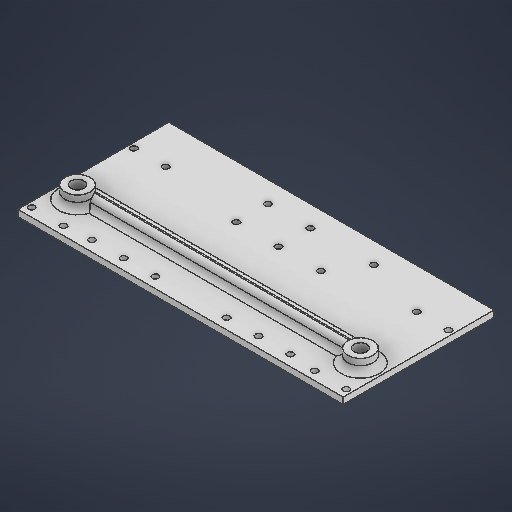
# Autodesk Inventor part: rigid_support1
Saved by Autodesk Inventor 2026.1 (Build 301233000, 233)
## iProperties
Created: 2025-10-27
Part Number: rigid_support1
Material: Generic
Document SubType Name: Modeling
Designer: emanuel
Density: 1 g/cm^3
Appearance: Default
Author: emanuel
Autodesk Inventor part; units mm, degrees
ref_plane "YZ Plane" through (0, 0, 0) normal (1, 0, 0) x (0, 1, 0)
ref_plane "XZ Plane" through (0, 0, 0) normal (0, 1, 0) x (-1, 0, 0)
ref_plane "XY Plane" through (0, 0, 0) normal (0, 0, 1) x (1, 0, 0)
sketch "Sketch1" plane through (0, 0, 0) normal (0, 1, 0) x (-1, 0, 0)
  line L0 (0, 0) -> (15, 0)
  line L1 (15, 0) -> (15, -48.3)
  line L2 (15, -48.3) -> (0, -48.3)
  line L3 (0, -48.3) -> (0, 0)
  circle A0 centre (15, 0) radius 1.5
  circle A1 centre (0, 0) radius 1.5
  circle A2 centre (15, -48.3) radius 1.5
  circle A3 centre (0, -48.3) radius 1.5
  line L4 (15, 0) -> (17.5, 0)
  line L5 (17.5, 0) -> (17.5, 4)
  line L6 (17.5, 4) -> (15, 4)
  line L7 (15, 4) -> (15, 0)
  line L8 (0, -48.3) -> (-2.5, -48.3)
  line L9 (-2.5, -48.3) -> (-2.5, -52.3)
  line L10 (-2.5, -52.3) -> (0, -52.3)
  line L11 (0, -52.3) -> (0, -48.3)
  line L12 (-2.5, -52.3) -> (17.5, -52.3)
  line L13 (17.5, -52.3) -> (17.5, 4)
  line L14 (17.5, 4) -> (-2.5, 4)
  line L15 (-2.5, 4) -> (-2.5, -52.3)
  line L16 (17.5, -26) -> (17.5, 4)
  line L17 (17.5, -44.8) -> (17.5, 4)
  line L18 (-2.5, -52.3) -> (-59.35, -52.3)
  line L19 (-2.5, -44.8) -> (-2.5, -52.3)
  line L20 (-2.5, 4) -> (-59.35, 4)
  line L21 (-59.35, 4) -> (-59.35, -52.3)
  line L22 (-59.35, -52.3) -> (-2.5, -52.3)
  line L23 (-2.5, -52.3) -> (-2.5, 4)
  line L24 (-118.7, 0) -> (-133.7, 0)
  line L25 (-133.7, 0) -> (-133.7, -48.3)
  line L26 (-133.7, -48.3) -> (-118.7, -48.3)
  line L27 (-118.7, -48.3) -> (-118.7, 0)
  circle A4 centre (-133.7, 0) radius 1.5
  circle A5 centre (-118.7, 0) radius 1.5
  circle A6 centre (-133.7, -48.3) radius 1.5
  circle A7 centre (-118.7, -48.3) radius 1.5
  line L28 (-133.7, 0) -> (-136.2, 0)
  line L29 (-136.2, 0) -> (-136.2, 4)
  line L30 (-136.2, 4) -> (-133.7, 4)
  line L31 (-133.7, 4) -> (-133.7, 0)
  line L32 (-118.7, -48.3) -> (-116.2, -48.3)
  line L33 (-116.2, -48.3) -> (-116.2, -52.3)
  line L34 (-116.2, -52.3) -> (-118.7, -52.3)
  line L35 (-118.7, -52.3) -> (-118.7, -48.3)
  line L36 (-116.2, -52.3) -> (-136.2, -52.3)
  line L37 (-136.2, -52.3) -> (-136.2, 4)
  line L38 (-136.2, 4) -> (-116.2, 4)
  line L39 (-116.2, 4) -> (-116.2, -52.3)
  line L40 (-136.2, -26) -> (-136.2, 4)
  line L41 (-136.2, -44.8) -> (-136.2, 4)
  line L42 (-116.2, -52.3) -> (-59.35, -52.3)
  line L43 (-116.2, -44.8) -> (-116.2, -52.3)
  line L44 (-116.2, 4) -> (-59.35, 4)
  line L45 (-59.35, -52.3) -> (-116.2, -52.3)
  line L46 (-116.2, -52.3) -> (-116.2, 4)
  point P0 (0, -52.3)
  point P1 (16.5, 0)
  point P2 (15, 1.5)
  dimension "d0" = 15
  dimension "d1" = 48.3
  dimension "d2" = 3
  dimension "d3" = 3
  dimension "d4" = 3
  dimension "d5" = 3
  dimension "d6" = 2.5
  dimension "d7" = 4
  dimension "d8" = 2.5
  dimension "d9" = 4
  dimension "d87" = 56.85
  constraints: 94 end point, 20 symmetric about line, 10 parallel, 8 centre point, 8 coincident, 6 horizontal, 5 perpendicular, 4 other
  measures "d0" distance of L1.end L2.end
  measures "d1" distance of L0.end L1.end
  measures "d2" diameter of A0
  measures "d3" diameter of A1
  measures "d4" diameter of A2
  measures "d5" diameter of A3
  measures "d6" distance of L6.end L5.end
  measures "d7" distance of L5.end L4.end
  measures "d8" distance of L10.end L9.end
  measures "d9" distance of L9.end L8.end
  measures "d87" distance of L9.end L18.end
extrude "Extrusion1" add sketch "Sketch1" along normal blind 3 contours A1 L3 A3 L8 L15 L14 L7 A0 L0 | L0 A0 L1 A2 L2 A3 L3 A1 | L7 L6 L5 L4 A0 | A0 L4 L13 L12 L11 A3 L2 A2 L1 | A3 L11 L10 L9 L8 | L9 L18 L21 L20 L15 | L21 L42 L33 L39 L44 | L39 L32 A7 L27 A5 L24 A4 L31 L38 | L34 L35 A7 L32 L33 | L31 A4 L28 L29 L30 | L36 L37 L28 A4 L25 A6 L26 A7 L35 | L24 A5 L27 A7 L26 A6 L25 A4
sketch "Sketch4" plane through (0, 3, 0) normal (0, 1, 0) x (1, 0, 0)
  line L0 (-17.5, -4) -> (-7.5, -4)
  line L1 (-7.5, -4) -> (-7.5, 14.15)
  line L2 (-7.5, 14.15) -> (-17.5, 14.15)
  line L3 (-17.5, 14.15) -> (-17.5, -4)
  circle A0 centre (-7.5, 14.15) radius 3.1
  line L4 (-17.5, 22.25) -> (-17.5, 17.25)
  line L5 (-17.5, -4) -> (136.2, -4) projected
  line L6 (136.2, -4) -> (126.2, -4)
  line L7 (126.2, -4) -> (126.2, 14.15)
  line L8 (126.2, 14.15) -> (136.2, 14.15)
  line L9 (136.2, 14.15) -> (136.2, -4)
  circle A1 centre (126.2, 14.15) radius 3.1
  circle A2 centre (-7.5, 14.15) radius 6
  circle A3 centre (126.2, 14.15) radius 6
  line L10 (-1.5, 14.15) -> (120.2, 14.15)
  line L11 (-7.5, 20.15) -> (126.2, 20.15)
  point P0 (0, 0)
  dimension "d54" = 10
  dimension "d55" = 18.15
  dimension "d60" = 6.2
  dimension "d89" = 10
  dimension "d90" = 18.15
  dimension "d91" = 6.2
  dimension "d92" = 12
  dimension "d93" = 12
  constraints: 22 end point, 4 centre point, 4 coincident, 4 parallel, 4 point on circle, 2 horizontal, 2 perpendicular, 1 tangent
  measures "d54" distance of L2.end L1.end
  measures "d55" distance of L1.end L0.end
  measures "d60" diameter of A0
  measures "d89" distance of L7.end L8.end
  measures "d90" distance of L6.end L7.end
  measures "d91" diameter of A1
  measures "d92" diameter of A2
  measures "d93" diameter of A3
extrude "Extrusion4" add sketch "Sketch4" along normal blind 6 contours A2 L2 A0 L1 | L1 A0 L2 A2 | A3 L8 A1 L7 | L7 A1 L8 A3
extrude "Extrusion6" add sketch "Sketch4" along normal blind 4 contours A2 L11 A3 L10
fillet "Fillet7" radius 3 7 edges at (59.35, 3, -20.15) (130.4426, 3, -18.3926) (126.2, 3, -8.15) (-11.7426, 3, -9.9074) (59.35, 3, -14.15) (59.35, 7, -20.15) (59.35, 7, -14.15)
sketch "Sketch6" plane through (0, 3, 0) normal (0, 1, 0) x (1, 0, 0)
  line L0 (136.2, 52.3) -> (-17.5, 52.3) projected
  line L1 (136.2, 52.3) -> (-17.5, 52.3)
  line L2 (-17.5, 52.3) -> (-17.5, 67.3)
  line L3 (-17.5, 67.3) -> (136.2, 67.3)
  line L4 (136.2, 67.3) -> (136.2, 52.3)
  point P0 (0, 0)
  point P1 (-17.5, 52.3)
  dimension "d97" = 15
  dimension "d137" = 153.7
  constraints: 8 end point, 2 parallel, 1 horizontal, 1 perpendicular
  measures "d97" distance of L1.end L2.end
  measures "d137" distance of L2.end L3.end
extrude "Extrusion7" add sketch "Sketch6" against normal blind 3
sketch "Sketch7" plane through (0, 3, 0) normal (0, 1, 0) x (1, 0, 0)
  line L0 (136.2, -4) -> (106.2, -4)
  line L1 (-17.5, -4) -> (136.2, -4) projected
  line L2 (106.2, -4) -> (106.2, 1)
  line L3 (106.2, 1) -> (91.2, 1)
  line L4 (91.2, 1) -> (76.2, 1)
  line L5 (-17.5, -4) -> (12.5, -4)
  line L6 (12.5, -4) -> (12.5, 1)
  line L7 (12.5, 1) -> (27.5, 1)
  line L8 (27.5, 1) -> (42.5, 1)
  line L9 (136.2, 67.3) -> (-17.5, 67.3) projected
  line L10 (59.35, 67.3) -> (59.35, 57.3)
  line L11 (59.35, 57.3) -> (69.35, 57.3)
  line L12 (69.35, 57.3) -> (49.35, 57.3)
  line L13 (49.35, 57.3) -> (49.35, 42.3)
  line L14 (49.35, 42.3) -> (69.35, 42.3)
  line L15 (69.35, 42.3) -> (69.35, 57.3)
  line L16 (69.35, 57.3) -> (89.35, 57.3)
  line L17 (89.35, 57.3) -> (89.35, 42.3)
  line L18 (89.35, 42.3) -> (69.35, 42.3)
  line L19 (69.35, 42.3) -> (69.35, 57.3)
  line L20 (49.35, 57.3) -> (29.35, 57.3)
  line L21 (29.35, 57.3) -> (29.35, 42.3)
  line L22 (29.35, 42.3) -> (49.35, 42.3)
  line L23 (49.35, 42.3) -> (49.35, 57.3)
  circle A0 centre (89.35, 57.3) radius 1.5
  circle A1 centre (79.35, 42.3) radius 1.5
  circle A2 centre (59.35, 42.3) radius 1.5
  circle A3 centre (59.35, 57.3) radius 1.5
  circle A4 centre (39.35, 57.3) radius 1.5
  circle A5 centre (39.35, 42.3) radius 1.5
  circle A6 centre (42.5, 1) radius 1.5
  circle A7 centre (27.5, 1) radius 1.5
  circle A8 centre (12.5, 1) radius 1.5
  line L24 (79.35, 42.3) -> (79.35, 57.3)
  circle A9 centre (79.35, 57.3) radius 1.5
  circle A10 centre (69.35, 57.3) radius 1.5
  circle A11 centre (69.35, 42.3) radius 1.5
  circle A12 centre (49.35, 42.3) radius 1.5
  circle A13 centre (49.35, 57.3) radius 1.5
  circle A14 centre (29.35, 57.3) radius 1.5
  circle A15 centre (29.35, 42.3) radius 1.5
  circle A16 centre (89.35, 42.3) radius 1.5
  circle A17 centre (106.2, 1) radius 1.5
  circle A18 centre (91.2, 1) radius 1.5
  circle A19 centre (76.2, 1) radius 1.5
  point P0 (0, 0)
  dimension "d104" = 30
  dimension "d105" = 5
  dimension "d106" = 15
  dimension "d107" = 15
  dimension "d109" = 30
  dimension "d110" = 5
  dimension "d111" = 15
  dimension "d112" = 15
  dimension "d113" = 10
  dimension "d114" = 10
  dimension "d115" = 20
  dimension "d116" = 15
  dimension "d117" = 20
  dimension "d118" = 15
  dimension "d119" = 20
  dimension "d120" = 15
  dimension "d121" = 3
  dimension "d122" = 3
  dimension "d123" = 3
  dimension "d124" = 3
  dimension "d125" = 3
  dimension "d126" = 3
  dimension "d132" = 3
  dimension "d133" = 3
  dimension "d134" = 3
  dimension "d138" = 3
  dimension "d139" = 3
  dimension "d140" = 3
  dimension "d141" = 3
  dimension "d142" = 3
  dimension "d143" = 3
  dimension "d144" = 3
  dimension "d145" = 3
  dimension "d146" = 3
  dimension "d147" = 3
  dimension "d148" = 3
  constraints: 46 end point, 20 centre point, 8 perpendicular, 6 parallel, 3 horizontal, 3 point on line, 2 midpoint, 1 coincident, 1 vertical
  measures "d104" distance of L0.start L0.end
  measures "d105" distance of L0.end L2.end
  measures "d106" distance of L2.end L3.end
  measures "d107" distance of L3.end L4.end
  measures "d109" distance of L1.start L5.end
  measures "d110" distance of L5.end L6.end
  measures "d111" distance of L6.end L7.end
  measures "d112" distance of L7.end L8.end
  measures "d113" distance of L10.start L10.end
  measures "d114" distance of L10.end L11.end
  measures "d115" distance of L14.end L13.end
  measures "d116" distance of L13.end L12.end
  measures "d117" distance of L17.end L18.end
  measures "d118" distance of L16.end L17.end
  measures "d119" distance of L22.end L21.end
  measures "d120" distance of L21.end L20.end
  measures "d121" diameter of A0
  measures "d122" diameter of A1
  measures "d123" diameter of A2
  measures "d124" diameter of A3
  measures "d125" diameter of A4
  measures "d126" diameter of A5
  measures "d132" diameter of A6
  measures "d133" diameter of A7
  measures "d134" diameter of A8
  measures "d138" diameter of A9
  measures "d139" diameter of A10
  measures "d140" diameter of A11
  measures "d141" diameter of A12
  measures "d142" diameter of A13
  measures "d143" diameter of A14
  measures "d144" diameter of A15
  measures "d145" diameter of A16
  measures "d146" diameter of A17
  measures "d147" diameter of A18
  measures "d148" diameter of A19
extrude "Extrusion8" cut sketch "Sketch7" against normal blind 3 contours A17 L3 L2 | L2 L3 A17 | A18 L4 L3 | L3 L4 A18 | A8 L7 L6 | L6 L7 A8 | A7 L8 L7 | L7 L8 A7 | A3 L11 L10 | L10 L12 A3 | L11 A3 L12 | A4 L20 | L20 A4 | A0 L17 L16 | L16 L17 A0 | L24 L18 A1 | A1 L18 L24 | L18 A1 | A2 L14 | L14 A2 | A5 L22 | L22 A5 | A6 | A19
body "Solid1"
